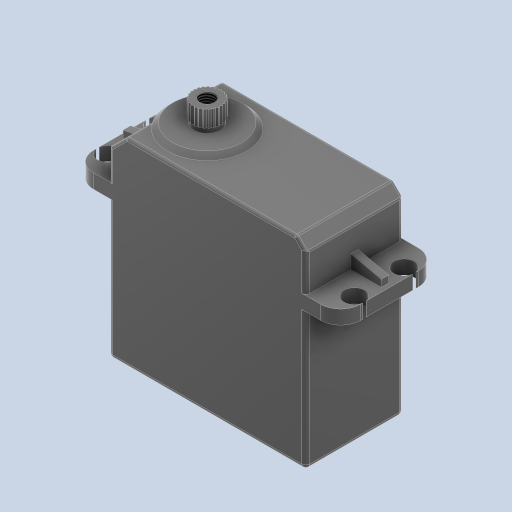
# Autodesk Inventor part: DSS_M1S_Servo
Saved by Autodesk Inventor 2023 (Build 270158000, 158)
## iProperties
Created: 2022-08-10
Part Number: DSS_M1S_Servo
Material: Thermoplastic Resin
Document SubType Name: Modeling
Designer: Windows10
Density: 1.28 g/cm^3
Appearance: Smooth - Black
Author: Windows10
Autodesk Inventor part; units mm, degrees
ref_plane "YZ Plane" through (0, 0, 0) normal (1, 0, 0) x (0, 1, 0)
ref_plane "XZ Plane" through (0, 0, 0) normal (0, 1, 0) x (-1, 0, 0)
ref_plane "XY Plane" through (0, 0, 0) normal (0, 0, 1) x (1, 0, 0)
sketch "Sketch1" plane through (0, 0, 0) normal (0, 0, 1) x (1, 0, 0)
  line L0 (0, 0) -> (39.6, 0)
  line L1 (39.6, 0) -> (39.6, 39.9)
  line L2 (39.6, 39.9) -> (0, 39.9)
  line L3 (0, 39.9) -> (0, 0)
  line L4 (19.8, 30.5) -> (-7, 30.5)
  line L5 (-7, 30.5) -> (-7, 27.7)
  line L6 (-7, 27.7) -> (19.8, 27.7)
  line L7 (19.8, 27.7) -> (19.8, 30.5)
  line L8 (19.8, 30.5) -> (19.8, 33.548)
  line L9 (19.8, 30.5) -> (46.6, 30.5)
  line L10 (46.6, 30.5) -> (46.6, 27.7)
  line L11 (46.6, 27.7) -> (19.8, 27.7)
  point P0 (0, 30.5)
  point P1 (0, 27.7)
  point P2 (39.6, 27.7)
  point P3 (39.6, 30.5)
  dimension "d0" = 39.6
  dimension "d1" = 39.9
  dimension "d2" = 26.8
  dimension "d3" = 2.8
  dimension "d4" = 27.7
  constraints: 24 end point, 4 parallel, 2 horizontal, 2 perpendicular, 2 symmetric about line, 1 vertical
  measures "d0" distance of L2.end L1.end
  measures "d1" distance of L1.end L0.end
  measures "d2" distance of L6.end L5.end
  measures "d3" distance of L4.end L5.end
  measures "d4" distance between parallel lines of L0 L6
extrude "Extrusion1" add sketch "Sketch1" along normal blind 19.6
chamfer "Chamfer1" distance 3.5 angle 45 1 edges at (0, 39.9, 9.8)
chamfer "Chamfer2" distance 2 angle 45 1 edges at (39.6, 39.9, 9.8)
ref_plane "Work Plane1" through (0, 0, 9.8) normal (0, 0, 1) x (1, 0, 0)
sketch "Sketch2" plane through (0, 0, 9.8) normal (0, 0, 1) x (1, 0, 0)
  line L0 (0, 30.5) -> (-7, 30.5) projected
  line L1 (-6.1508, 30.5) -> (-6.1508, 31.9055)
  line L2 (-6.1508, 31.9055) -> (0, 33.2772)
  line L3 (0, 36.4) -> (0, 30.5) projected
  line L4 (37.6, 39.9) -> (3.5, 39.9) projected
  line L5 (20.55, 39.9) -> (21.3491, 36.4)
  line L6 (19.8, -0.261) -> (19.8, 1.5705)
  line L7 (39.6, 30.5) -> (46.6, 30.5)
  line L8 (45.7508, 30.5) -> (45.7508, 31.9055)
  line L9 (45.7508, 31.9055) -> (39.6, 33.2772)
  line L10 (39.6, 30.5) -> (39.6, 37.9) projected
  point P0 (0, 0)
  constraints: 14 end point, 5 symmetric about line, 3 point on line, 2 vertical, 1 midpoint
extrude "Extrusion2" add sketch "Sketch2" along normal mid plane 1.5
fillet "Fillet2" radius 0.8 12 edges at (0, 13.85, 19.6) (0, 13.85, 0) (39.6, 13.85, 19.6) (0, 33.45, 19.6) (39.6, 34.2, 19.6) (0, 33.45, 0) (39.6, 34.2, 0) (39.6, 13.85, 0) (19.8, 0, 0) (19.8, 0, 19.6) (0, 0, 9.8) (39.6, 0, 9.8)
fillet "Fillet3" radius 0.5 10 edges at (20.55, 39.9, 19.6) (20.55, 39.9, 0) (2.15, 38.55, 19.6) (2.15, 38.55, 0) (38.2, 39.3, 19.6) (38.2, 39.3, 0) (3.5, 39.9, 9.8) (37.6, 39.9, 9.8) (39.6, 37.9, 9.8) (0, 36.4, 9.8)
sketch "Sketch3" plane through (-6.1508, 30.5, 10.55) normal (0, 1, 0) x (1, 0, 0)
  circle A0 centre (50.7008, 5.75) radius 2.075
  line L0 (63.5058, 0.75) -> (-11.6042, 0.75) projected
  circle A1 centre (50.7008, -4.25) radius 2.075
  line L1 (6.9508, -8.25) -> (44.9508, -8.25) projected
  line L2 (25.9508, -8.25) -> (25.9508, -11.4131)
  circle A2 centre (1.2008, 5.75) radius 2.075
  circle A3 centre (1.2008, -4.25) radius 2.075
  line L3 (-0.8492, 10.55) -> (-0.8492, -9.05) projected
  line L4 (52.7508, 10.55) -> (52.7508, -9.05) projected
  line L5 (52.7508, 10.55) -> (44.9508, 10.55) projected
  point P0 (6.1508, 10.55)
  dimension "d19" = 4.15
  dimension "d20" = 5
  dimension "d21" = 49.5
  dimension "d67" = 53.6
  dimension "d68" = 2.05
  dimension "d69" = 4.8
  constraints: 4 centre point, 3 symmetric about line, 2 end point, 1 midpoint, 1 vertical, 3 other
  measures "d19" diameter of A0
  measures "d20" distance from line of L0 A0.centre
  measures "d21" distance of A2.centre A0.centre
  measures "d67" distance between parallel lines of L3 L4
  measures "d68" distance from line of L4 A0.centre
  measures "d69" distance from line of L5 A0.centre
extrude "Extrusion3" cut sketch "Sketch3" against normal blind 7.5
fillet "Fillet1" radius 4 4 edges at (-7, 29.1, 19.6) (-7, 29.1, 0) (46.6, 29.1, 19.6) (46.6, 29.1, 0)
sketch "Sketch4" plane through (3.7071, 39.9, 0.5) normal (0, 1, 0) x (1, 0, 0)
  circle A0 centre (6.2929, -9.3) radius 2.9
  line L0 (-3.7071, -0.3) -> (-3.7071, -18.3) projected
  line L1 (33.6858, 0.5) -> (0, 0.5) projected
  circle A1 centre (6.2929, -9.3) radius 2.65
  line L2 (6.2929, -9.3) -> (6.2929, -8.1563)
  circle A2 centre (6.2929, -9.3) radius 1.5
  line L3 (5.9608, -6.6709) -> (6.3304, -6.4002)
  line L4 (6.625, -6.6709) -> (6.3304, -6.4002)
  line L5 (5.3174, -6.8361) -> (5.6081, -6.482)
  line L6 (5.9608, -6.6709) -> (5.6081, -6.482)
  line L7 (4.7353, -7.1561) -> (4.9288, -6.7408)
  line L8 (5.3174, -6.8361) -> (4.9288, -6.7408)
  line L9 (4.251, -7.6108) -> (4.3352, -7.1605)
  line L10 (4.7353, -7.1561) -> (4.3352, -7.1605)
  line L11 (3.8951, -8.1717) -> (3.8647, -7.7145)
  line L12 (4.251, -7.6108) -> (3.8647, -7.7145)
  line L13 (3.6898, -8.8034) -> (3.5467, -8.3682)
  line L14 (3.8951, -8.1717) -> (3.5467, -8.3682)
  line L15 (3.6481, -9.4664) -> (3.4012, -9.0805)
  line L16 (3.6898, -8.8034) -> (3.4012, -9.0805)
  line L17 (3.7726, -10.1189) -> (3.4375, -9.8065)
  line L18 (3.6481, -9.4664) -> (3.4375, -9.8065)
  line L19 (4.0554, -10.7199) -> (3.6531, -10.5007)
  line L20 (3.7726, -10.1189) -> (3.6531, -10.5007)
  line L21 (4.4788, -11.2318) -> (4.0347, -11.1194)
  line L22 (4.0554, -10.7199) -> (4.0347, -11.1194)
  line L23 (5.0162, -11.6222) -> (4.5581, -11.6239)
  line L24 (4.4788, -11.2318) -> (4.5581, -11.6239)
  line L25 (5.6339, -11.8667) -> (5.1905, -11.9823)
  line L26 (5.0162, -11.6222) -> (5.1905, -11.9823)
  line L27 (6.2929, -11.95) -> (5.8922, -12.1722)
  line L28 (5.6339, -11.8667) -> (5.8922, -12.1722)
  line L29 (6.9519, -11.8667) -> (6.6191, -12.1816)
  line L30 (6.2929, -11.95) -> (6.6191, -12.1816)
  line L31 (7.5695, -11.6222) -> (7.3255, -12.0099)
  line L32 (6.9519, -11.8667) -> (7.3255, -12.0099)
  line L33 (8.1069, -11.2318) -> (7.967, -11.668)
  line L34 (7.5695, -11.6222) -> (7.967, -11.668)
  line L35 (8.5304, -10.7199) -> (8.5033, -11.1773)
  line L36 (8.1069, -11.2318) -> (8.5033, -11.1773)
  line L37 (8.8132, -10.1189) -> (8.9007, -10.5686)
  line L38 (8.5304, -10.7199) -> (8.9007, -10.5686)
  line L39 (8.9377, -9.4664) -> (9.1343, -9.8802)
  line L40 (8.8132, -10.1189) -> (9.1343, -9.8802)
  line L41 (8.896, -8.8034) -> (9.1893, -9.1554)
  line L42 (8.9377, -9.4664) -> (9.1893, -9.1554)
  line L43 (8.6907, -8.1717) -> (9.0623, -8.4396)
  line L44 (8.896, -8.8034) -> (9.0623, -8.4396)
  line L45 (8.3348, -7.6108) -> (8.7614, -7.7779)
  line L46 (8.6907, -8.1717) -> (8.7614, -7.7779)
  line L47 (7.8505, -7.1561) -> (8.3053, -7.2119)
  line L48 (8.3348, -7.6108) -> (8.3053, -7.2119)
  line L49 (7.2684, -6.8361) -> (7.7228, -6.777)
  line L50 (7.8505, -7.1561) -> (7.7228, -6.777)
  line L51 (6.625, -6.6709) -> (7.0504, -6.5007)
  line L52 (7.2684, -6.8361) -> (7.0504, -6.5007)
  point P0 (-3.7071, 0.5)
  point P1 (6.2929, -6.65)
  dimension "d26" = 5.8
  dimension "d24" = 10
  dimension "d25" = 9.8
  dimension "d31" = 0.25
  dimension "d32" = 3
  dimension "d36" = 360
  constraints: 102 end point, 3 point on circle, 2 centre point, 2 coincident, 1 symmetric about line, 1 vertical, 129 other
  measures "d24" distance from line of L0 L2.start
  measures "d25" distance from line of L1 L2.start
  measures "d32" diameter of A2
extrude "Extrusion5" add sketch "Sketch4" along normal blind 2 contours A1
sketch "Sketch5" plane through (10, 41.9, 9.8) normal (0, 1, 0) x (1, 0, 0)
  circle A0 centre (0, 0) radius 2.65 projected
  line L0 (-6.2929, 9.3) -> (27.3929, 9.3) projected
  line L1 (-6.2929, -9.3) -> (-6.2929, 9.3) projected
  line L2 (27.3929, -9.3) -> (-6.2929, -9.3) projected
  line L3 (27.3929, 9.3) -> (27.3929, -9.3) projected
  circle A1 centre (0, 0) radius 2.9
  line L4 (-3.707, -0.3) -> (-3.707, -18.3)
  line L5 (33.6858, 0.5) -> (0, 0.5)
  circle A2 centre (0, 0) radius 2.65
  line L6 (0, 0) -> (0, 1.1437)
  circle A3 centre (0, 0) radius 1.5
  line L7 (-0.3321, 2.6291) -> (0.0375, 2.8998)
  line L8 (0.3321, 2.6291) -> (0.0375, 2.8998)
  line L9 (-0.9755, 2.4639) -> (-0.6848, 2.818)
  line L10 (-0.3321, 2.6291) -> (-0.6848, 2.818)
  line L11 (-1.5576, 2.1439) -> (-1.3641, 2.5592)
  line L12 (-0.9755, 2.4639) -> (-1.3641, 2.5592)
  line L13 (-2.0419, 1.6892) -> (-1.9577, 2.1395)
  line L14 (-1.5576, 2.1439) -> (-1.9577, 2.1395)
  line L15 (-2.3978, 1.1283) -> (-2.4282, 1.5855)
  line L16 (-2.0419, 1.6892) -> (-2.4282, 1.5855)
  line L17 (-2.6031, 0.4966) -> (-2.7462, 0.9318)
  line L18 (-2.3978, 1.1283) -> (-2.7462, 0.9318)
  line L19 (-2.6448, -0.1664) -> (-2.8917, 0.2195)
  line L20 (-2.6031, 0.4966) -> (-2.8917, 0.2195)
  line L21 (-2.5203, -0.8189) -> (-2.8554, -0.5065)
  line L22 (-2.6448, -0.1664) -> (-2.8554, -0.5065)
  line L23 (-2.2375, -1.4199) -> (-2.6398, -1.2007)
  line L24 (-2.5203, -0.8189) -> (-2.6398, -1.2007)
  line L25 (-1.814, -1.9318) -> (-2.2582, -1.8194)
  line L26 (-2.2375, -1.4199) -> (-2.2582, -1.8194)
  line L27 (-1.2766, -2.3222) -> (-1.7348, -2.3239)
  line L28 (-1.814, -1.9318) -> (-1.7348, -2.3239)
  line L29 (-0.659, -2.5667) -> (-1.1024, -2.6823)
  line L30 (-1.2766, -2.3222) -> (-1.1024, -2.6823)
  line L31 (0, -2.65) -> (-0.4007, -2.8722)
  line L32 (-0.659, -2.5667) -> (-0.4007, -2.8722)
  line L33 (0.659, -2.5667) -> (0.3262, -2.8816)
  line L34 (0, -2.65) -> (0.3262, -2.8816)
  line L35 (1.2766, -2.3222) -> (1.0326, -2.7099)
  line L36 (0.659, -2.5667) -> (1.0326, -2.7099)
  line L37 (1.814, -1.9318) -> (1.6741, -2.368)
  line L38 (1.2766, -2.3222) -> (1.6741, -2.368)
  line L39 (2.2375, -1.4199) -> (2.2104, -1.8773)
  line L40 (1.814, -1.9318) -> (2.2104, -1.8773)
  line L41 (2.5203, -0.8189) -> (2.6078, -1.2686)
  line L42 (2.2375, -1.4199) -> (2.6078, -1.2686)
  line L43 (2.6448, -0.1664) -> (2.8414, -0.5802)
  line L44 (2.5203, -0.8189) -> (2.8414, -0.5802)
  line L45 (2.6031, 0.4966) -> (2.8964, 0.1446)
  line L46 (2.6448, -0.1664) -> (2.8964, 0.1446)
  line L47 (2.3978, 1.1283) -> (2.7694, 0.8604)
  line L48 (2.6031, 0.4966) -> (2.7694, 0.8604)
  line L49 (2.0419, 1.6892) -> (2.4685, 1.5221)
  line L50 (2.3978, 1.1283) -> (2.4685, 1.5221)
  line L51 (1.5576, 2.1439) -> (2.0124, 2.0881)
  line L52 (2.0419, 1.6892) -> (2.0124, 2.0881)
  line L53 (0.9755, 2.4639) -> (1.4299, 2.523)
  line L54 (1.5576, 2.1439) -> (1.4299, 2.523)
  line L55 (0.3321, 2.6291) -> (0.7575, 2.7993)
  line L56 (0.9755, 2.4639) -> (0.7575, 2.7993)
  point P0 (-10, 9.8)
  point P1 (-3.7071, 0.5)
  point P2 (0, 2.65)
  dimension "d42" = 5.8
  dimension "d40" = 3.707
  dimension "d41" = 0.5
  dimension "d43" = 0.25
  dimension "d44" = 3
  dimension "d45" = 360
  dimension "d46" = 1.15
  constraints: 106 end point, 3 point on circle, 2 centre point, 2 coincident, 1 symmetric about line, 1 vertical, 129 other
  measures "d40" distance from line of L4 L6.start
  measures "d41" distance from line of L5 L6.start
  measures "d44" diameter of A3
  measures "d46" radial gap between concentric circles of A3 A2
extrude "Extrusion6" add sketch "Sketch5" along normal blind 3.3 contours A0 | A0 L9 L10
pattern_circular "Circular Pattern1" [suppressed]
pattern_circular "Circular Pattern2" count 25 over 360 about axis through (10, 39.9, 9.8) along (0, 1, 0) of "Extrusion6"
thread "Thread1" size "M3x0.5" class "6H" standard "ANSI Metric M Profile" full length
sketch "Sketch6" plane through (0, 0.8, 18.8) normal (-1, 0, 0) x (0, 0, 1)
  line L0 (-12.0463, 8.7721) -> (-5.9537, 8.7721)
  line L1 (-5.9537, 8.7721) -> (-5.9537, 6.6046)
  line L2 (-5.9537, 6.6046) -> (-12.0463, 6.6046)
  line L3 (-12.0463, 6.6046) -> (-12.0463, 8.7721)
  point P0 (-18.8, -0.8)
  point P1 (-9, 7.6884)
  point P2 (-12.0463, 7.6884)
  point P3 (-9, 8.7721)
  constraints: 8 end point, 2 midpoint, 2 parallel, 1 horizontal, 1 horizontal alignment, 1 perpendicular, 1 vertical alignment
extrude "Extrusion7" add sketch "Sketch6" along normal blind 2.75 separate body
fillet "Fillet4" radius 0.5 4 edges at (-1.375, 9.5721, 12.8463) (-1.375, 7.4046, 12.8463) (-1.375, 9.5721, 6.7537) (-1.375, 7.4046, 6.7537)
sketch "Sketch7" plane through (3.7071, 39.9, 0.5) normal (0, 1, 0) x (1, 0, 0)
  circle A0 centre (6.2929, -9.3) radius 1.5 projected
  circle A1 centre (6.2929, -9.3) radius 7.9233
  point P0 (-3.7071, 0.5)
  constraints: 1 centre point, 1 coincident
extrude "cable extrusion" add sketch "Sketch7" along normal blind 1 and the other way blind 3.75 bodies 1
chamfer "Chamfer3" distance 1 angle 45 1 edges at (2.0767, 40.9, 9.8)
body "Solid1"
